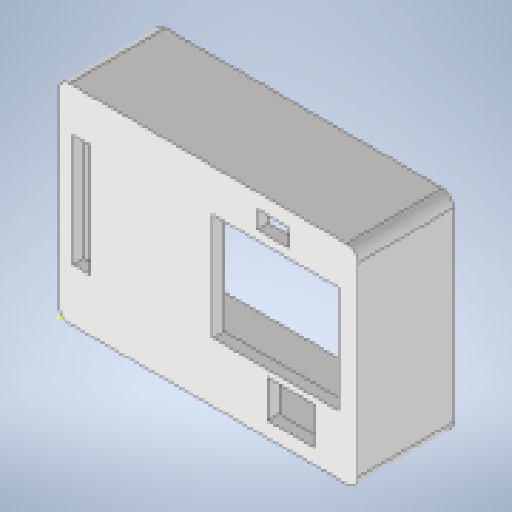
# Autodesk Inventor part: Frame_Lid
Saved by Autodesk Inventor 2023 (Build 270158000, 158)
## iProperties
Created: 2023-10-08
Part Number: Frame_Lid
Material: Generic
Document SubType Name: Modeling
Designer: a laptop
Density: 1 g/cm^3
Appearance: Default
Author: a laptop
Autodesk Inventor part; units mm, degrees
ref_plane "YZ Plane" through (0, 0, 0) normal (1, 0, 0) x (0, 1, 0)
ref_plane "XZ Plane" through (0, 0, 0) normal (0, 1, 0) x (-1, 0, 0)
ref_plane "XY Plane" through (0, 0, 0) normal (0, 0, 1) x (1, 0, 0)
sketch "Sketch1" plane through (0, 0, 0) normal (0, 0, 1) x (1, 0, 0)
  line L0 (2, 0) -> (51.18, 0)
  line L1 (53.18, 2) -> (53.18, 34.924)
  line L2 (51.18, 36.924) -> (2, 36.924)
  line L3 (0, 34.924) -> (0, 2)
  arc A0 (2, 36.924) -> (0, 34.924) centre (2, 34.924) ccw
  arc A1 (0, 2) -> (2, 0) centre (2, 2) ccw
  arc A2 (51.18, 0) -> (53.18, 2) centre (51.18, 2) ccw
  arc A3 (53.18, 34.924) -> (51.18, 36.924) centre (51.18, 34.924) ccw
  point P0 (0, 0)
  point P1 (53.18, 36.924)
  point P2 (53.18, 0)
  point P3 (0, 36.924)
  dimension "d0" = 36.924
  dimension "d1" = 53.18
  dimension "d2" = 2
  constraints: 8 end point, 8 point on circle, 8 point on line, 8 tangent, 4 centre point, 3 equal radius, 2 parallel, 1 horizontal, 1 perpendicular
  measures "d0" distance of point (53.18, 0) point (53.18, 36.924)
  measures "d1" distance of point (53.18, 36.924) point (0, 36.924)
  measures "d2" radius of A0
extrude "Extrusion1" add sketch "Sketch1" along normal blind 2
sketch "Sketch2" plane through (0, 0, 2) normal (0, 0, 1) x (1, 0, 0)
  point P0 (0, 0)
sketch "Sketch3" plane through (0, 0, 2) normal (0, 0, 1) x (1, 0, 0)
  line L0 (3.9641, 27.5862) -> (4.2577, 27.5862) projected
  line L1 (4.2577, 27.5862) -> (4.2577, 27.8798) projected
  line L2 (4.2577, 27.8798) -> (3.9641, 27.8798) projected
  line L3 (3.9641, 27.8798) -> (3.9641, 27.5862) projected
  line L4 (3.9793, 10.8373) -> (4.2425, 10.8373) projected
  line L5 (4.2425, 10.8373) -> (4.2425, 11.1006) projected
  line L6 (4.2425, 11.1006) -> (3.9793, 11.1006) projected
  line L7 (3.9793, 11.1006) -> (3.9793, 10.8373) projected
  line L8 (2.5409, 9.399) -> (5.6809, 9.399)
  line L9 (5.6809, 9.399) -> (5.6809, 29.303)
  line L10 (5.6809, 29.303) -> (2.5409, 29.303)
  line L11 (2.5409, 29.303) -> (2.5409, 9.399)
  line L12 (36.7302, 32.8328) -> (36.7302, 32.5392) projected
  line L13 (36.7302, 32.5392) -> (37.0238, 32.5392) projected
  line L14 (37.0238, 32.5392) -> (37.0238, 32.8328) projected
  line L15 (37.0238, 32.8328) -> (36.7302, 32.8328) projected
  line L16 (39.2702, 32.8328) -> (39.2702, 32.5392) projected
  line L17 (39.2702, 32.5392) -> (39.5638, 32.5392) projected
  line L18 (39.5638, 32.5392) -> (39.5638, 32.8328) projected
  line L19 (39.5638, 32.8328) -> (39.2702, 32.8328) projected
  line L20 (35.307, 34.256) -> (40.987, 34.256)
  line L21 (40.987, 34.256) -> (40.987, 31.116)
  line L22 (40.987, 31.116) -> (35.307, 31.116)
  line L23 (35.307, 31.116) -> (35.307, 34.256)
  arc A0 (51.18, 0) -> (53.18, 2) centre (51.18, 2) ccw projected
  line L24 (53.18, 2) -> (53.18, 34.924) projected
  arc A1 (53.18, 34.924) -> (51.18, 36.924) centre (51.18, 34.924) ccw projected
  line L25 (51.18, 36.924) -> (2, 36.924) projected
  arc A2 (2, 36.924) -> (0, 34.924) centre (2, 34.924) ccw projected
  line L26 (0, 34.924) -> (0, 2) projected
  arc A3 (0, 2) -> (2, 0) centre (2, 2) ccw projected
  line L27 (2, 0) -> (51.18, 0) projected
  line L28 (49.341, 10.949) -> (27.8799, 10.949) construction
  line L29 (27.8799, 10.949) -> (27.8799, 21.149) construction
  line L30 (27.8799, 21.149) -> (49.341, 21.149) construction
  line L31 (49.341, 21.149) -> (49.341, 10.949) construction
  line L32 (49.741, 10.549) -> (27.4799, 10.549)
  line L33 (27.4799, 10.549) -> (27.4799, 21.549)
  line L34 (27.4799, 21.549) -> (49.741, 21.549) construction
  line L35 (49.741, 21.549) -> (49.741, 10.549)
  line L36 (49.741, 21.549) -> (27.4799, 21.549) construction
  line L37 (27.4799, 21.549) -> (27.4799, 29.0699)
  line L38 (27.4799, 29.0699) -> (49.741, 29.0699) construction
  line L39 (49.741, 29.0699) -> (49.741, 21.549)
  line L40 (27.4799, 29.0699) -> (49.741, 29.0699)
  line L41 (49.741, 29.0699) -> (49.741, 29.4699)
  line L42 (49.741, 29.4699) -> (27.4799, 29.4699)
  line L43 (27.4799, 29.4699) -> (27.4799, 29.0699)
  line L44 (37.1719, 9.3139) -> (45.4719, 9.3139)
  line L45 (45.4719, 9.3139) -> (45.4719, 2.7139)
  line L46 (45.4719, 2.7139) -> (37.1719, 2.7139)
  line L47 (37.1719, 2.7139) -> (37.1719, 9.3139)
  point P0 (0, 0)
  point P1 (3.9793, 10.969)
  point P2 (4.1109, 11.1006)
  point P3 (4.1109, 9.399)
  point P4 (4.1109, 29.303)
  point P5 (3.9641, 27.733)
  point P6 (36.877, 32.8328)
  point P7 (39.417, 32.8328)
  point P8 (39.5638, 32.686)
  point P9 (40.987, 32.686)
  point P10 (27.8799, 11.076)
  point P11 (27.883, 21.5699)
  point P12 (49.304, 29.0699)
  point P13 (49.304, 21.5699)
  point P14 (27.883, 29.0699)
  point P15 (37.5719, 8.9139)
  point P16 (45.0719, 3.1139)
  dimension "d5" = 1.57
  dimension "d6" = 1.57
  dimension "d7" = 1.57
  dimension "d8" = 1.57
  dimension "d9" = 1.57
  dimension "d10" = 1.57
  dimension "d13" = 0.4
  dimension "d14" = 0.4
  dimension "d15" = 0.4
  dimension "d16" = 0.4
  dimension "d17" = 0.4
  dimension "d18" = 0.4
  dimension "d19" = 0.4
  dimension "d20" = 0.4
  dimension "d21" = 0.4
  constraints: 56 end point, 14 parallel, 9 midpoint, 7 horizontal, 7 perpendicular, 5 point on line, 1 horizontal alignment, 1 vertical alignment, 9 other
  measures "d5" distance from line of L8 point (3.979, 10.969)
  measures "d6" distance from line of L11 point (4.111, 11.101)
  measures "d7" vertical distance of point (4.111, 29.303) point (3.964, 27.733)
  measures "d8" distance from line of L23 point (36.877, 32.833)
  measures "d9" distance from line of L21 point (39.417, 32.833)
  measures "d10" distance from line of L20 point (39.564, 32.686)
  measures "d13" distance between parallel lines of L28 L32
  measures "d14" distance between parallel lines of L30 L34
  measures "d15" distance between parallel lines of L33 L29
  measures "d16" distance between parallel lines of L35 L31
  measures "d17" distance between parallel lines of L40 L42
  measures "d18" distance from line of L44 point (37.572, 8.914)
  measures "d19" distance from line of L47 point (37.572, 8.914)
  measures "d20" distance from line of L46 point (45.072, 3.114)
  measures "d21" distance from line of point (45.072, 3.114) L45
extrude "Extrusion2" cut sketch "Sketch3" against normal through all contours L3 L2 L1 L0 | L7 L6 L5 L4 | L11 L10 L9 L8 | L15 L14 L13 L12 | L19 L18 L17 L16 | L20 L21 L22 L23 | L32 L33 L37 L40 L39 L35 | L40 L43 L42 L41 | L44 L45 L46 L47
sketch "Sketch4" plane through (0, 0, 0) normal (0, 0, -1) x (-1, 0, 0)
  arc A0 (-2, 0) -> (0, 2) centre (-2, 2) ccw projected
  line L0 (0, 2) -> (0, 34.924) projected
  line L1 (-51.18, 0) -> (-2, 0) projected
  arc A1 (-53.18, 2) -> (-51.18, 0) centre (-51.18, 2) ccw projected
  line L2 (-53.18, 34.924) -> (-53.18, 2) projected
  arc A2 (-51.18, 36.924) -> (-53.18, 34.924) centre (-51.18, 34.924) ccw projected
  line L3 (-2, 36.924) -> (-51.18, 36.924) projected
  arc A3 (0, 34.924) -> (-2, 36.924) centre (-2, 34.924) ccw projected
  point P0 (0, 0)
extrude "Extrusion3" add sketch "Sketch4" along normal blind 15 separate body
shell "Shell1" thickness 1.6 removed faces 3 at (12.9473, 16.417, 0) at (34.7867, 12.308, 0) at (34.7867, 12.308, -15) bodies 2
combine bodies "Combine1" operation type add bodies to combine 1 2
body "Solid2"
